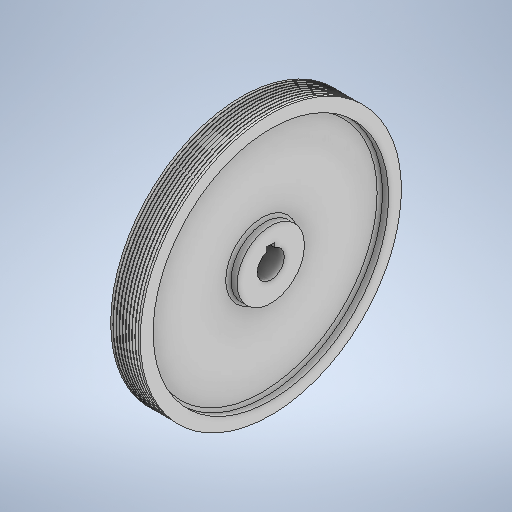
# Autodesk Inventor part: 29-10-201
Saved by Autodesk Inventor 2025.2 (Build 292293000, 293)
## iProperties
Created: 2024-11-29
Part Number: 29-10-201
Material: Generic
Document SubType Name: Modeling
Designer: Zvonko.Gabric
Density: 1 g/cm^3
Appearance: Default
Description: Polly-V pulley PJ8 22mm
Author: Zvonko.Gabric
Autodesk Inventor part; units mm, degrees
ref_plane "YZ Plane" through (0, 0, 0) normal (1, 0, 0) x (0, 1, 0)
ref_plane "XZ Plane" through (0, 0, 0) normal (0, 1, 0) x (-1, 0, 0)
ref_plane "XY Plane" through (0, 0, 0) normal (0, 0, 1) x (1, 0, 0)
sketch "Sketch1" plane through (0, 0, 0) normal (0, 1, 0) x (-1, 0, 0)
  line L0 (7.7855, 95.0028) -> (8.4486, 96.867)
  line L1 (6.4884, 96.867) -> (7.1825, 95.0028)
  arc A0 (8.8254, 96.867) -> (8.4486, 96.867) centre (8.637, 96.8) ccw
  arc A1 (6.4884, 96.867) -> (6.1115, 96.867) centre (6.3, 96.8) ccw
  arc A2 (4.8455, 95.0028) -> (5.4485, 95.0028) centre (5.147, 95.11) ccw
  arc A3 (9.5196, 95.0028) -> (10.1226, 95.0028) centre (9.8211, 95.11) ccw
  line L2 (8.8254, 96.867) -> (9.5196, 95.0028)
  line L3 (10.1226, 95.0028) -> (10.7856, 96.867)
  line L4 (4.1514, 96.867) -> (4.8455, 95.0028)
  arc A4 (11.1624, 96.867) -> (10.7856, 96.867) centre (10.974, 96.8) ccw
  arc A5 (4.1514, 96.867) -> (3.7745, 96.867) centre (3.963, 96.8) ccw
  line L5 (3.1115, 95.0028) -> (3.7745, 96.867)
  line L6 (11.1624, 96.867) -> (11.8566, 95.0028)
  arc A6 (2.5085, 95.0028) -> (3.1115, 95.0028) centre (2.81, 95.11) ccw
  arc A7 (11.8566, 95.0028) -> (12.4596, 95.0028) centre (12.1581, 95.11) ccw
  line L7 (12.4596, 95.0028) -> (13.1226, 96.867)
  line L8 (1.7649, 97) -> (2.5085, 95.0028)
  arc A8 (13.4995, 96.867) -> (13.1226, 96.867) centre (13.311, 96.8) ccw
  line L9 (13.4995, 96.867) -> (14.1936, 95.0028)
  line L10 (0, 97) -> (1.7649, 97)
  arc A9 (15.8365, 96.867) -> (15.4596, 96.867) centre (15.648, 96.8) ccw
  arc A10 (16.5306, 95.0028) -> (17.1336, 95.0028) centre (16.8321, 95.11) ccw
  line L11 (17.1336, 95.0028) -> (17.7966, 96.867)
  line L12 (18.1735, 96.867) -> (18.8676, 95.0028)
  arc A11 (18.8676, 95.0028) -> (19.4706, 95.0028) centre (19.1691, 95.11) ccw
  line L13 (19.4706, 95.0028) -> (20.1809, 97)
  line L14 (20.1809, 97) -> (22, 97)
  line L15 (0, 0) -> (0, 97)
  line L16 (22, 0) -> (0, 0)
  line L17 (22, 0) -> (0, 0)
  line L18 (22, 97) -> (22, 0)
  arc A12 (14.1936, 95.0028) -> (14.7966, 95.0028) centre (14.4951, 95.11) ccw
  line L19 (5.4485, 95.0028) -> (6.1115, 96.867)
  arc A13 (7.1825, 95.0028) -> (7.7855, 95.0028) centre (7.484, 95.11) ccw
  arc A14 (18.1735, 96.867) -> (17.7966, 96.867) centre (17.9851, 96.8) ccw
  line L20 (15.8365, 96.867) -> (16.5306, 95.0028)
  line L21 (14.7966, 95.0028) -> (15.4596, 96.867)
  dimension "d0" = 0
  dimension "d1" = 22
  dimension "d2" = 97
  dimension "d3" = 97
  dimension "d4" = 1.7649
  dimension "d5" = 90
  dimension "d6" = 40
  dimension "d7" = 40
  dimension "d8" = 40
  dimension "d9" = 40
  dimension "d10" = 40
  dimension "d11" = 40
  dimension "d12" = 40
  dimension "d13" = 40
  dimension "d14" = 1.8191
  dimension "d15" = 2.8309
  dimension "d16" = 4.0149
  dimension "d17" = 5.1679
  dimension "d18" = 6.352
  dimension "d19" = 7.5049
  dimension "d20" = 8.689
  dimension "d21" = 9.8419
  dimension "d22" = 11.026
  dimension "d23" = 12.179
  dimension "d24" = 13.363
  dimension "d25" = 14.516
  dimension "d26" = 15.7
  dimension "d27" = 16.853
  dimension "d28" = 2.81
  dimension "d29" = 3.9629
  dimension "d30" = 0.32
  dimension "d31" = 0.2
  dimension "d32" = 0.32
  dimension "d33" = 0.2
  dimension "d34" = 0.32
  dimension "d35" = 0.2
  dimension "d36" = 0.32
  dimension "d37" = 0.2
  dimension "d38" = 0.32
  dimension "d39" = 0.2
  dimension "d40" = 0.32
  dimension "d41" = 0.2
  dimension "d42" = 0.32
  dimension "d43" = 0.2
  dimension "d44" = 0.32
  dimension "d46" = 1.89
  dimension "d47" = 0.2
  dimension "d48" = 1.89
  dimension "d49" = 1.89
  dimension "d50" = 0.2
  dimension "d51" = 0.2
  dimension "d52" = 1.89
  dimension "d53" = 0.2
  dimension "d54" = 1.89
  dimension "d55" = 0.2
  dimension "d56" = 1.89
  dimension "d57" = 0.2
  dimension "d58" = 0.2
  dimension "d59" = 1.89
  dimension "d60" = 1.89
  dimension "d61" = 109.578
  dimension "d62" = 110.422
  constraints: 44 end point, 30 point on circle, 15 centre point
  measures "d0" distance of point (0, 0) L15.start
  measures "d1" distance of L16.start L15.start
  measures "d2" distance of L14.end L16.start
  measures "d3" distance of L15.start L10.start
  measures "d4" distance of L10.start L8.start
  measures "d5" angle of L10 L15
  measures "d6" angle of L5 L8
  measures "d7" angle of L19 L4
  measures "d8" angle of L0 L1
  measures "d9" angle of L3 L2
  measures "d10" angle of L7 L6
  measures "d11" angle of L21 L9
  measures "d12" angle of L11 L20
  measures "d13" angle of L13 L12
  measures "d14" distance of L13.end L14.end
  measures "d15" distance from line of L18 A11.centre
  measures "d16" distance from line of L18 A14.centre
  measures "d17" distance from line of L18 A10.centre
  measures "d18" distance from line of L18 A9.centre
  measures "d19" distance from line of L18 A12.centre
  measures "d20" distance from line of L18 A8.centre
  measures "d21" distance from line of L18 A7.centre
  measures "d22" distance from line of L18 A4.centre
  measures "d23" distance from line of L18 A3.centre
  measures "d24" distance from line of L18 A0.centre
  measures "d25" distance from line of L18 A13.centre
  measures "d26" distance from line of L18 A1.centre
  measures "d27" distance from line of L18 A2.centre
  measures "d28" distance from line of L15 A6.centre
  measures "d29" distance from line of L15 A5.centre
  measures "d30" radius of A6
  measures "d31" radius of A5
  measures "d32" radius of A2
  measures "d33" radius of A1
  measures "d34" radius of A13
  measures "d35" radius of A0
  measures "d36" radius of A3
  measures "d37" radius of A4
  measures "d38" radius of A7
  measures "d39" radius of A8
  measures "d40" radius of A12
  measures "d41" radius of A9
  measures "d42" radius of A10
  measures "d43" radius of A14
  measures "d44" radius of A11
  measures "d46" distance from line of L10 A6.centre
  measures "d47" distance from line of L10 A5.centre
  measures "d48" distance from line of L10 A2.centre
  measures "d49" distance from line of L10 A13.centre
  measures "d50" distance from line of L10 A1.centre
  measures "d51" distance from line of L10 A0.centre
  measures "d52" distance from line of L10 A3.centre
  measures "d53" distance from line of L10 A4.centre
  measures "d54" distance from line of L14 A7.centre
  measures "d55" distance from line of L14 A8.centre
  measures "d56" distance from line of L14 A12.centre
  measures "d57" distance from line of L14 A9.centre
  measures "d58" distance from line of L14 A14.centre
  measures "d59" distance from line of L14 A11.centre
  measures "d60" distance from line of L14 A10.centre
  measures "d61" angle of L13 L14
  measures "d62" angle of L8 L10
revolve "Revolution1" add sketch "Sketch1" angle 360 about axis through (-22, 0, 0) along (1, 0, 0)
sketch "Sketch2" plane through (0, 0, 0) normal (1, 0, 0) x (0, 0, -1)
  circle A0 centre (0, 0) radius 87.5
  circle A1 centre (0, 0) radius 25
  dimension "d63" = 175
  dimension "d64" = 50
  constraints: 2 centre point, 2 coincident
  measures "d63" diameter of A0
  measures "d64" diameter of A1
extrude "Extrusion1" cut sketch "Sketch2" against normal blind 6.5
sketch "Sketch3" plane through (-22, 0, 0) normal (-1, 0, 0) x (0, 0, 1)
  circle A0 centre (0, 0) radius 87.5
  circle A1 centre (0, 0) radius 25
  dimension "d67" = 175
  dimension "d68" = 50
  constraints: 2 centre point, 2 coincident
  measures "d67" diameter of A0
  measures "d68" diameter of A1
extrude "Extrusion2" cut sketch "Sketch3" against normal blind 6.5
fillet "Fillet1" radius 2 4 edges at (-6.5, 0, 87.5) (-6.5, 0, 25) (-15.5, 0, -25) (-15.5, 0, -87.5)
sketch "Sketch4" plane through (-22, 0, 0) normal (-1, 0, 0) x (0, 0, 1)
  arc A0 (-3, 9.5394) -> (3, 9.5394) centre (0, 0) ccw
  line L0 (0, 12.8) -> (-3, 12.8)
  line L1 (-3, 12.8) -> (-3, 9.5394)
  line L2 (0, 12.8) -> (3, 12.8)
  line L3 (3, 12.8) -> (3, 9.5394)
  point P0 (-1.5, 12.8)
  point P1 (0, 11.4)
  dimension "d72" = 20
  dimension "d73" = 12.8
  dimension "d75" = 0
  dimension "d76" = 6
  dimension "d79" = 3
  dimension "d80" = 3
  dimension "d81" = 3
  dimension "d82" = 12.8
  constraints: 8 end point, 2 point on circle, 1 centre point, 1 coincident, 1 midpoint, 1 perpendicular
  measures "d72" diameter of A0
  measures "d73" vertical distance of point (0, 0) point (-1.5, 12.8)
  measures "d75" horizontal distance of point (0, 0) point (0, 11.4)
  measures "d76" distance between parallel lines of L1 L3
  measures "d79" distance of L0.start L2.end
  measures "d80" distance of L0.start L0.end
  measures "d81" distance from line of point (0, 0) L1
  measures "d82" distance from line of point (0, 0) L0
extrude "Extrusion3" cut sketch "Sketch4" against normal blind 30
fillet "Fillet2" radius 0.2 2 edges at (-1.7649, 0, -97) (-20.1809, 0, -97)
body "Solid1"
